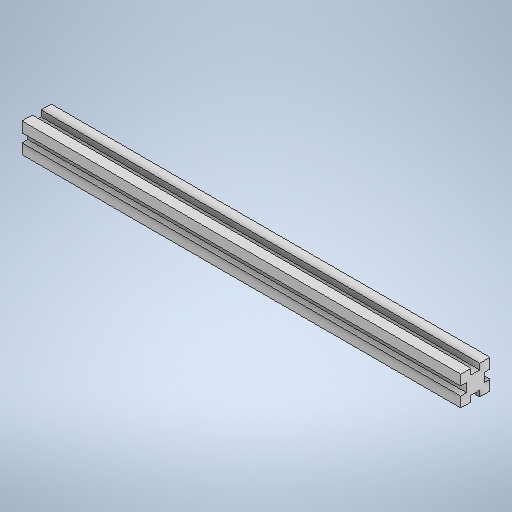
# Autodesk Inventor part: barre_horizontale_support_pinces
Saved by Autodesk Inventor 2025 (Build 290162000, 162)
## iProperties
Created: 2024-11-18
Part Number: barre_horizontale_support_pinces
Material: Générique
Document SubType Name: Modeling
Designer: chass
Density: 1 g/cm^3
Appearance: Par défaut
Author: chass
Autodesk Inventor part; units mm, degrees
ref_plane "YZ Plane" through (0, 0, 0) normal (1, 0, 0) x (0, 1, 0)
ref_plane "XZ Plane" through (0, 0, 0) normal (0, 1, 0) x (-1, 0, 0)
ref_plane "XY Plane" through (0, 0, 0) normal (0, 0, 1) x (1, 0, 0)
sketch "Esquisse1" plane through (0, 0, 0) normal (1, 0, 0) x (0, 1, 0)
  line L0 (10, 10) -> (-10, 10)
  line L1 (-10, 10) -> (-10, -10)
  line L2 (-10, -10) -> (10, -10)
  line L3 (10, -10) -> (10, 10)
  line L4 (10, 3) -> (6, 3)
  line L5 (6, 3) -> (6, -3)
  line L6 (6, -3) -> (10, -3)
  line L7 (10, -3) -> (10, 3)
  line L8 (0, 14.3918) -> (0, -21)
  line L9 (14, 0) -> (-15, 0)
  line L10 (-10, 3) -> (-6, 3)
  line L11 (-6, 3) -> (-6, -3)
  line L12 (-6, -3) -> (-10, -3)
  line L13 (-10, -3) -> (-10, 3)
  line L14 (3, 10) -> (-3, 10)
  line L15 (-3, 10) -> (-3, 6)
  line L16 (-3, 6) -> (3, 6)
  line L17 (3, 6) -> (3, 10)
  line L18 (3, -10) -> (-3, -10)
  line L19 (-3, -10) -> (-3, -6)
  line L20 (-3, -6) -> (3, -6)
  line L21 (3, -6) -> (3, -10)
  point P0 (0, 0)
  point P1 (3, 8)
  point P2 (3, -8)
  dimension "d0" = 20
  dimension "d1" = 6
  dimension "d2" = 4
  dimension "d3" = 6
  dimension "d4" = 4
  dimension "d5" = 3
  dimension "d6" = 0
  constraints: 44 end point, 9 symmetric about line, 6 parallel, 4 horizontal, 3 perpendicular, 2 point on line, 1 midpoint, 1 vertical
  measures "d0" distance of L1.end L2.end
  measures "d1" distance of L4.end L5.end
  measures "d2" distance of L4.start L4.end
  measures "d3" distance of L16.end L15.end
  measures "d4" distance of L15.end L14.end
  measures "d5" distance from line of L8 point (3, 8)
  measures "d6" distance from line of point (0, 0) L8
extrude "Extrusion1" add sketch "Esquisse1" along normal blind 300 contours L3 L4 L5 L9 L8 L16 L17 L0 | L15 L16 L8 L9 L11 L10 L1 L0 | L3 L2 L21 L20 L8 L9 L5 L6 | L8 L20 L19 L2 L1 L12 L11 L9
